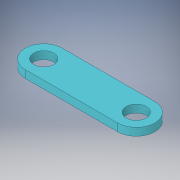
# Autodesk Inventor part: Middle_leg_b
Saved by Autodesk Inventor 2017 (Build 210142000, 142)
## iProperties
Created: 2016-06-08
Part Number: Middle_leg_b
Material: Generic
Document SubType Name: Modeling
Designer: alex-
Density: 1 g/cm^3
Appearance: Cadet Blue
Author: alex-
Autodesk Inventor part; units mm, degrees
ref_plane "YZ Plane" through (0, 0, 0) normal (1, 0, 0) x (0, 1, 0)
ref_plane "XZ Plane" through (0, 0, 0) normal (0, 1, 0) x (-1, 0, 0)
ref_plane "XY Plane" through (0, 0, 0) normal (0, 0, 1) x (1, 0, 0)
sketch "Sketch1" plane through (0, 0, 0) normal (0, 1, 0) x (-1, 0, 0)
  circle A0 centre (30, 0) radius 12
  circle A1 centre (-30, 0) radius 12
  line L0 (-30, 12) -> (30, 12)
  line L1 (-30, -12) -> (30, -12)
  circle A2 centre (30, 0) radius 6.5
  circle A3 centre (-30, 0) radius 6.5
  line L2 (58.8, 0) -> (-58.8, 0) projected
  line L3 (2.5, -9) -> (-2.5, -9)
  line L4 (-2.5, -9) -> (-2.5, -4)
  line L5 (-2.5, -4) -> (2.5, -4)
  line L6 (2.5, -4) -> (2.5, -9)
  line L7 (2.5, 9) -> (-2.5, 9)
  line L8 (-2.5, 9) -> (-2.5, 4)
  line L9 (-2.5, 4) -> (2.5, 4)
  line L10 (2.5, 4) -> (2.5, 9)
  point P0 (0, 0)
  point P1 (0, 12)
  point P2 (0, -9)
  dimension "d0" = 60
  dimension "d1" = 24
  dimension "d2" = 13
  dimension "d5" = 5
  dimension "d6" = 5
  dimension "d10" = 4
  constraints: 20 end point, 4 centre point, 4 point on circle, 4 symmetric about line, 4 tangent, 3 parallel, 2 coincident, 2 horizontal alignment, 2 midpoint, 2 vertical alignment, 1 equal radius, 1 horizontal, 1 perpendicular
  measures "d0" distance of A1.centre A0.centre
  measures "d1" diameter of A0
  measures "d2" diameter of A2
  measures "d5" distance of L3.start L3.end
  measures "d6" distance of L5.end L3.start
  measures "d10" distance between parallel lines of L2 L5
extrude "Extrusion2" add sketch "Sketch1" along normal blind 5 contours L2 A2 A0 | A0 L2 A2 | A0 L2 A1 L0 | L1 A1 L2 A0 | A1 L2 A3 | A1 L2 A3 | L3 L4 L5 L6 | L10 L9 L8 L7
equation "\"d1\" = sa_diameter"
equation "\"d2\" = bb_outer_diameter"
equation "\"d5\" = b_mat_thickness"
equation "\"d6\" = b_mat_thickness"
equation "\"d10\" = 0.8 * b_mat_thickness"
equation "\"d8\" = b_mat_thickness"
equation "\"sa_diameter\" = 24"
equation "\"bb_outer_diameter\" = 13"
equation "\"b_mat_thickness\" = 5"
body "Solid2"
